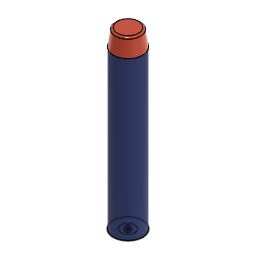
Nerf Dart (Autodesk Fusion 360 design; units mm, degrees)
Autodesk Fusion 360 part; units mm, degrees
sketch "Sketch1" plane through (0, 0, 0) normal (0, 0, 1) x (1, 0, 0)
  circle A0 centre (0, 0) radius 6
  circle A1 centre (0, 0) radius 2.8
  dimension "d1" = 12
  dimension "d4" = -3.2
  constraint coincident A0.centre A1.centre
  measures "d1" diameter of A0
sketch "Sketch2" plane through (0, 0, 72) normal (0, 0, 1) x (1, 0, 0)
  circle A0 centre (0, 0) radius 6
  circle A1 centre (0, 0) radius 5
  dimension "d5" = 10
  constraint concentric A0 A1
  measures "d5" diameter of A1
extrude "Extrude1" add sketch "Sketch1" along normal blind 65 contours A0 | A1 makes body 1
extrude "Extrude2" cut sketch "Sketch1" along normal up to surface (55 mm away) contours A1 bodies 1
loft "Loft1" add profiles "Sketch2" section 1 face at (-0.9566, -0.2914, 65) section 2 contours A1 separate body on bodies 1 makes body 2
fillet "Fillet1" radius 0.8 1 edges at (-4.6616, 1.8081, 72) on bodies 2
